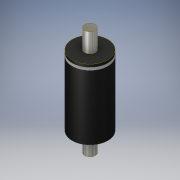
# Autodesk Inventor part: 1N4007
Saved by Autodesk Inventor 2017 (Build 210142000, 142)
## iProperties
Part Number: 1N4007
Material: Generisch
Document SubType Name: Modeling
Designer: Philomena-Theresa
Density: 1 g/cm^3
Appearance: Vorgabe
Author: Philomena-Theresa
Autodesk Inventor part; units mm, degrees
ref_plane "YZ Plane" through (0, 0, 0) normal (1, 0, 0) x (0, 1, 0)
ref_plane "XZ Plane" through (0, 0, 0) normal (0, 1, 0) x (-1, 0, 0)
sketch "Skizze1" plane through (0, 0, 0) normal (0, 0, 1) x (1, 0, 0)
  circle A0 centre (0, 0) radius 1.3
  dimension "d0" = 2.6
  constraints: 1 centre point, 1 coincident
  measures "d0" diameter of A0
extrude "Extrusion1" add sketch "Skizze1" along normal mid plane 4.7
sketch "Skizze4" plane through (0, 0, 2.35) normal (0, 0, 1) x (1, 0, 0)
  circle A0 centre (0, 0) radius 1.3
  constraints: 1 centre point, 1 coincident
extrude "Extrusion4" add sketch "Skizze4" along normal blind 0.2 separate body
sketch "Skizze5" plane through (0, 0, 2.55) normal (0, 0, 1) x (1, 0, 0)
  circle A0 centre (0, 0) radius 1.3
  constraints: 1 centre point, 1 coincident
extrude "Extrusion5" add sketch "Skizze5" along normal blind 0.2 separate body
sketch "Skizze6" plane through (0, 0, 2.75) normal (0, 0, 1) x (1, 0, 0)
  circle A0 centre (0, 0) radius 0.39
  dimension "d13" = 0.78
  constraints: 1 centre point, 1 coincident
  measures "d13" diameter of A0
extrude "Extrusion6" add sketch "Skizze6" along normal blind 1.4 bodies 3
ref_plane "Arbeitsebene1" through (0, 0, 0.2) normal (0, 0, 1) x (1, 0, 0)
mirror "Spiegeln1" about plane through (0, 0, 0.2) normal (0, 0, 1) of "Extrusion6" bodies 3
ref_plane "Arbeitsebene2" through (0, 0, 0.2) normal (0, 0, 1) x (1, 0, 0)
